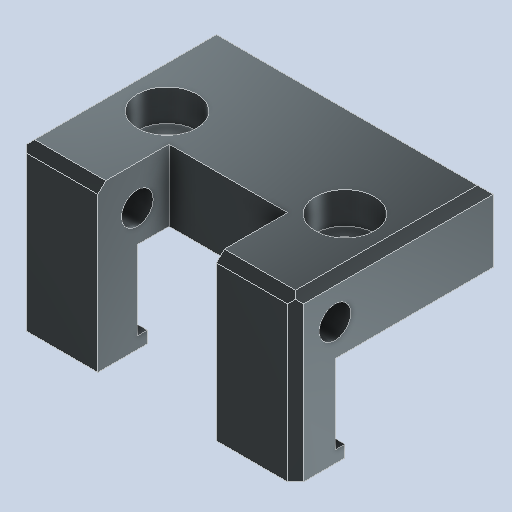
# Autodesk Inventor part: Lager
Saved by Autodesk Inventor 2024.1 (Build 281209000, 209)
## iProperties
Created: 2023-05-11
Part Number: Lager
Material: Iron, Cast
Document SubType Name: Modeling
Designer: Raj
Density: 7.15 g/cm^3
Appearance: Iron Gray
Author: Raj
Autodesk Inventor part; units mm, degrees
ref_plane "YZ Plane" through (0, 0, 0) normal (1, 0, 0) x (0, 1, 0)
ref_plane "XZ Plane" through (0, 0, 0) normal (0, 1, 0) x (-1, 0, 0)
ref_plane "XY Plane" through (0, 0, 0) normal (0, 0, 1) x (1, 0, 0)
sketch "Sketch1" plane through (0, 0, 0) normal (0, 0, 1) x (1, 0, 0)
  line L0 (35, 25) -> (-35, 25)
  line L1 (-35, 25) -> (-35, -25)
  line L2 (-35, -25) -> (35, -25)
  line L3 (35, -25) -> (35, 25)
  line L4 (35, 25) -> (-35, -25) construction
  line L5 (-35, 25) -> (35, -25) construction
  point P0 (0, 0)
  dimension "d0" = 70
  dimension "d1" = 50
  constraints: 12 end point, 2 midpoint, 2 parallel, 1 horizontal, 1 perpendicular
  measures "d0" distance of L2.end L1.end
  measures "d1" distance of L1.end L0.end
extrude "Extrusion1" add sketch "Sketch1" along normal blind 41
sketch "Sketch2" plane through (-35, -25, 0) normal (-1, 0, 0) x (0, 0, 1)
  line L0 (0, 50) -> (23, 50)
  line L1 (0, 50) -> (41, 50) projected
  line L2 (23, 50) -> (23, 10)
  line L3 (23, 10) -> (3, 10)
  line L4 (3, 10) -> (3, 12.5)
  line L5 (3, 12.5) -> (0, 12.5)
  line L6 (0, 0) -> (41, 0) projected
  line L7 (0, 50) -> (0, 12.5)
  point P0 (0, 25)
  dimension "d4" = 23
  dimension "d5" = 40
  dimension "d6" = 20
  dimension "d7" = 12.5
  constraints: 12 end point, 5 perpendicular, 1 point on line
  measures "d4" distance of L0.start L0.end
  measures "d5" distance of L0.end L2.end
  measures "d6" distance of L2.end L3.end
  measures "d7" distance between parallel lines of L6 L5
extrude "Extrusion2" cut sketch "Sketch2" against normal through all
sketch "Sketch3" plane through (0, 0, 41) normal (0, 0, 1) x (1, 0, 0)
  line L0 (-15, -7) -> (15, -7)
  line L1 (15, -7) -> (15, -25)
  line L2 (15, -25) -> (-15, -25)
  line L3 (-15, -25) -> (-15, -7)
  line L4 (-35, -25) -> (35, -25) projected
  point P0 (0, 0)
  dimension "d10" = 30
  dimension "d11" = 18
  dimension "d12" = 15
  dimension "d13" = 0
  constraints: 8 end point, 2 parallel, 1 horizontal, 1 perpendicular
  measures "d10" distance of L1.end L2.end
  measures "d11" distance of L0.end L1.end
  measures "d12" distance from line of point (0, 0) L1
  measures "d13" distance between parallel lines of L4 L2
extrude "Extrusion3" cut sketch "Sketch3" against normal through all
sketch "Sketch4" plane through (0, 0, 41) normal (0, 0, 1) x (1, 0, 0)
  line L0 (35, 25) -> (-35, 25) projected
  point P0 (0, 0)
  point P1 (-22.5, 0)
  point P2 (22.5, 0)
  dimension "d16" = 25
  dimension "d17" = 22.5
  dimension "d18" = 45
  dimension "d19" = 25
  measures "d16" distance from line of point (-22.5, 0) L0
  measures "d17" distance of point (-22.5, 0) point (0, 0)
  measures "d18" distance of point (-22.5, 0) point (22.5, 0)
  measures "d19" distance from line of point (22.5, 0) L0
hole "Hole1" at (-22.5, 0, 41) at (22.5, 0, 41) direction (0, 0, -1) diameter 8.4 end through all counterbore diameter 15 counterbore depth 8
sketch "Sketch5" plane through (-35, -25, 41) normal (-1, 0, 0) x (0, 0, 1)
  line L0 (0, 50) -> (0, 0) projected
  line L1 (-41, 0) -> (0, 0) projected
  point P0 (-41, 25)
  point P1 (-10, 10)
  dimension "d27" = 10
  dimension "d28" = 10
  measures "d27" distance from line of point (-10, 10) L0
  measures "d28" distance from line of point (-10, 10) L1
hole "Hole2" at (-35, -15, 31) direction (1, 0, 0) diameter 8 end through all
chamfer "Chamfer1" distance 2 angle 45 7 edges at (-35, 0, 41) (-25, -25, 41) (0, 25, 41) (35, 0, 41) (25, -25, 41) (-35, -25, 20.5) (35, -25, 20.5)
body "Solid1"
